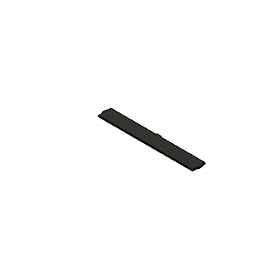
006_nixie_top_plate (Autodesk Fusion 360 design; units mm, degrees)
Autodesk Fusion 360 part; units mm, degrees
note: some values were not read from the file. Set by a fixed rule: which sketch regions a step uses.
sketch "Sketch1" plane through (0, 114.5, 0) normal (0, 1, 0) x (-1, 0, 0)
  line L0 (-255, -14) -> (-205, -14) construction
  line L1 (-205, -14) -> (-205, -13) construction
  line L2 (-205, -13) -> (-255, -13) construction
  line L3 (-255, -13) -> (-255, -14) construction
  line L4 (-205, -14) -> (-200, -14) construction
  line L5 (-200, -14) -> (-200, -13) construction
  line L6 (-200, -13) -> (-205, -13) construction
  line L7 (-205, -13) -> (-205, -14) construction
  line L8 (-200, -14) -> (-150, -14) construction
  line L9 (-150, -14) -> (-150, -13) construction
  line L10 (-150, -13) -> (-200, -13) construction
  line L11 (-200, -13) -> (-200, -14) construction
  line L12 (-255, -9) -> (-255, -4) construction
  line L13 (-255, -4) -> (-256, -4) construction
  line L14 (-256, -4) -> (-256, -9) construction
  line L15 (-256, -9) -> (-255, -9) construction
  line L16 (-720, 0) -> (0, 0) construction
  line L17 (0, 0) -> (0, 2) construction
  line L18 (0, 2) -> (-720, 2) construction
  line L19 (-720, 2) -> (-720, 0) construction
  line L20 (-150, -4) -> (-150, -9) construction
  line L21 (-150, -9) -> (-149, -9) construction
  line L22 (-149, -9) -> (-149, -4) construction
  line L23 (-149, -4) -> (-150, -4) construction
  line L24 (-255, -9) -> (-256, -9)
  line L25 (-256, -9) -> (-256, -4)
  line L26 (-256, -4) -> (-255, -4)
  line L27 (-150, -9) -> (-149, -9)
  line L28 (-149, -9) -> (-149, -4)
  line L29 (-149, -4) -> (-150, -4)
  line L30 (-200, -13) -> (-200, -14)
  line L31 (-200, -14) -> (-205, -14)
  line L32 (-205, -14) -> (-205, -13)
  line L33 (-150, -9) -> (-150, -13)
  line L34 (-255, -13) -> (-255, -9)
  line L35 (-150, -13) -> (-200, -13)
  line L36 (-205, -13) -> (-255, -13)
  line L37 (-255, 0) -> (-150, 0) construction
  line L38 (-150, 0) -> (-150, 2) construction
  line L39 (-150, 2) -> (-255, 2) construction
  line L40 (-255, 2) -> (-255, 0) construction
  line L41 (-150, 1) -> (-255, 1)
  line L42 (-150, -4) -> (-150, 1)
  line L43 (-255, -4) -> (-255, 1)
  constraint horizontal L35
  constraint vertical L34
  constraint coincident L9.end L10.start
  constraint horizontal L24
  constraint vertical L25
  constraint horizontal L26
  constraint coincident L13.end L14.start
  constraint coincident L12.start L15.end
  constraint horizontal L27
  constraint vertical L28
  constraint horizontal L29
  constraint coincident L22.end L23.start
  constraint coincident L20.end L21.start
  constraint vertical L30
  constraint horizontal L31
  constraint vertical L32
  constraint coincident L4.end L5.start
  constraint coincident L1.end L2.start
  constraint collinear L3 L34
  constraint collinear L35 L36
  constraint coincident L12.end L13.start
  constraint coincident L5.end L6.start
  constraint coincident L38 L41.start
  constraint midpoint L40 L41.end
  constraint coincident L38.end L39.start
  constraint midpoint L38 L41.start
  constraint coincident L20.start L23.end
extrude "Extrude1" add sketch "Sketch1" against normal blind 1
